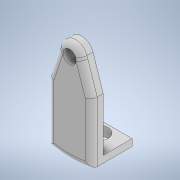
# Autodesk Inventor part: Tool Head Clamp
Saved by Autodesk Inventor 2022.2 (Build 262287000, 287)
## iProperties
Created: 2022-08-16
Part Number: Tool Head Clamp
Material: Generic
Document SubType Name: Modeling
Designer: Ilewicz
Density: 1 g/cm^3
Appearance: Default
Author: Ilewicz
Autodesk Inventor part; units mm, degrees
ref_plane "YZ Plane" through (0, 0, 0) normal (1, 0, 0) x (0, 1, 0)
ref_plane "XZ Plane" through (0, 0, 0) normal (0, 1, 0) x (-1, 0, 0)
ref_plane "XY Plane" through (0, 0, 0) normal (0, 0, 1) x (1, 0, 0)
sketch "Sketch1" plane through (0, 0, 0) normal (0, 0, 1) x (1, 0, 0)
  circle A0 centre (0, 8.95) radius 1.09 projected
  arc A1 (1.662, 7.8375) -> (-0.0143, 6.9501) centre (0, 8.95) ccw projected
  arc A2 (1.8983, 9.5797) -> (-1.8983, 9.5797) centre (0, 8.95) ccw
  line L0 (3.6, 4.45) -> (3.6, -5.6116)
  arc A3 (-3.6, -5.6116) -> (3.6, -5.6116) centre (0, 8.95) ccw
  circle A4 centre (0, 8.95) radius 4.08 projected
  circle A5 centre (0, 8.95) radius 15 projected
  line L1 (2.5, -0.05) -> (2.5, 4.45) projected
  line L2 (2.5, 4.45) -> (3.6, 4.45) projected
  line L3 (3.6, 4.45) -> (3.6, -4.45) projected
  line L4 (3.6, -4.45) -> (-3.6, -4.45) projected
  line L5 (-3.6, -4.45) -> (-3.6, 4.45) projected
  line L6 (-3.6, 4.45) -> (-2.5, 4.45) projected
  line L7 (-2.5, 4.45) -> (-2.5, -0.05) projected
  line L8 (-3.6, -5.6116) -> (-3.6, 4.45)
  line L9 (-3.6, 4.45) -> (-1.8983, 9.5797)
  line L10 (3.6, 4.45) -> (1.8983, 9.5797)
  line L11 (-2.5, -0.05) -> (2.5, -0.05) projected
  point P0 (0, 0)
  point P1 (-1.8983, 9.5797)
  constraints: 8 end point, 6 point on circle, 3 tangent, 2 centre point, 2 collinear, 1 concentric
extrude "Extrusion1" add sketch "Sketch1" along normal blind 2 contours L10 A4 L9 A1 | L10 L2 L1 L11 L7 L6 L9 A4 | L0 L4 L5 L6 L7 L11 L1 L2 | L0 A3 L8 L4 picked at (1.9915, 8.1578)
sketch "Sketch2" plane through (0, 0, 0) normal (0, 0, -1) x (-1, 0, 0)
  line L0 (-3.6, -4.45) -> (3.6, -4.45) projected
  line L1 (-3.6, 4.45) -> (-1.8983, 9.5797) projected
  line L2 (-3.6, -5.6116) -> (-3.6, 4.45) projected
  arc A0 (-3.6, -5.6116) -> (3.6, -5.6116) centre (0, 8.95) ccw projected
  line L3 (3.6, 4.45) -> (3.6, -5.6116) projected
  line L4 (1.8983, 9.5797) -> (3.6, 4.45) projected
  arc A1 (1.8983, 9.5797) -> (-1.8983, 9.5797) centre (0, 8.95) ccw projected
  circle A2 centre (0, 8.95) radius 1.09 projected
  point P0 (0, 0)
ref_plane "Work Plane1" through (-15.2152, -6.2652, -4.8) normal (0, 0, 1) x (1, 0, 0)
extrude "Extrusion2" add sketch "Sketch2" along normal up to surface (4.8 mm away) contours L0 L3 A0 L2
sketch "Sketch3" plane through (-3.6, -4.45, 0) normal (0, 1, 0) x (1, 0, 0)
  circle A0 centre (3.6, 2.8) radius 1.6 projected
  point P0 (3.6, 0)
extrude "Extrusion3" cut sketch "Sketch3" against normal blind 10
fillet "Fillet1" radius 1 6 edges at (2.7491, 7.0149, 2) (3.6, -0.5808, 2) (0, -6.05, 2) (-3.6, -0.5808, 2) (-2.7491, 7.0149, 2) (0, 10.95, 2)
body "Solid1"
